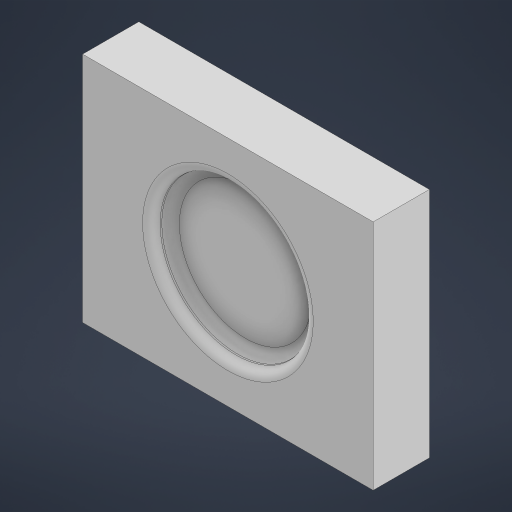
# Autodesk Inventor part: stanzev1u
Saved by Autodesk Inventor 2024.3 (Build 283343010, 343A)
## iProperties
Created: 2025-05-07
Part Number: stanzev1u
Material: Generisch
Document SubType Name: Modeling
Designer: David
Density: 1 g/cm^3
Appearance: Vorgabe
Author: David
## iProperties of the stored document stanzev1u_3D-Druck.ipt
Created: 2025-05-07
Part Number: stanzev1u_3D-Druck
Material: Generisch
Document SubType Name: Modeling
Designer: David
Density: 1 g/cm^3
Appearance: Vorgabe
Author: David
Autodesk Inventor part; units mm, degrees
ref_plane "YZ Plane" through (0, 0, 0) normal (1, 0, 0) x (0, 1, 0)
ref_plane "XZ Plane" through (0, 0, 0) normal (0, 1, 0) x (-1, 0, 0)
ref_plane "XY Plane" through (0, 0, 0) normal (0, 0, 1) x (1, 0, 0)
sketch "Skizze1" plane through (0, 0, 0) normal (0, 0, 1) x (1, 0, 0)
  line L0 (0, 0) -> (3.5, 0)
  line L1 (3.5, 0) -> (3.6763, 1)
  line L2 (3.6763, 1) -> (11.3237, 1)
  line L3 (11.3237, 1) -> (11.5, 0)
  line L4 (11.5, 0) -> (15, 0)
  line L5 (15, 0) -> (15, -3)
  line L6 (15, -3) -> (0, -3)
  line L7 (0, -3) -> (0, 0)
  line L8 (3.5, 0) -> (7.5, 0)
  line L9 (7.5, 0) -> (7.5, 1)
  line L10 (11.4076, 1.1) -> (3.5924, 1.1)
  line L11 (3.5924, 1.1) -> (3.4161, 0.1)
  line L12 (3.4161, 0.1) -> (0, 0.1)
  line L13 (15, 0.1) -> (11.5839, 0.1)
  line L14 (11.5839, 0.1) -> (11.4076, 1.1)
  line L15 (0, 0) -> (0, 3)
  line L16 (0, 3) -> (15, 3)
  line L17 (15, 0) -> (15, 3)
  line L18 (7.5, 0) -> (11.5, 0)
  line L19 (7.5, 1) -> (7.5, 1.1)
  line L20 (3.4161, 0.1) -> (11.5839, 0.1)
  dimension "d0" = 3
  dimension "d1" = 15
  dimension "d2" = 8
  dimension "d3" = 10
  dimension "d4" = 0.1
  dimension "d5" = 1
  dimension "d6" = 0.1
  dimension "d7" = 3
  constraints: 42 end point, 6 point on line, 5 perpendicular, 2 equal length, 2 horizontal, 2 midpoint, 2 parallel, 1 vertical, 3 other
  measures "d0" distance of L6.end L0.start
  measures "d1" distance of L5.end L6.end
  measures "d2" diameter of L0.end L9
  measures "d3" angle of L9 L1
  measures "d4" distance between parallel lines of L2 L10
  measures "d5" distance between parallel lines of L0 L2
  measures "d6" distance between parallel lines of L4 L13
  measures "d7" distance of L0.start L15.end
extrude "Extrusion1" add sketch "Skizze1" along normal mid plane 12 contours L15 L16 L17 L13 L14 L10 L11 L12 | L20 L11 L10 L19 L2 L1 | L1 L2 L9 L20 | L9 L2 L3 L20 | L19 L10 L14 L20 L3 L2
revolve "Umdrehung1" cut sketch "Skizze1" angle 360 about axis through (7.5, 0, 0) along (0, 1, 0) contours L1 L20 L9 L8 | L1 L2 L9 L20
fillet "Rundung1" radius 0.5 2 edges at (11.3237, 1, 0) (11.4824, 0.1, 0)
equation "\"d6\" = d4"
